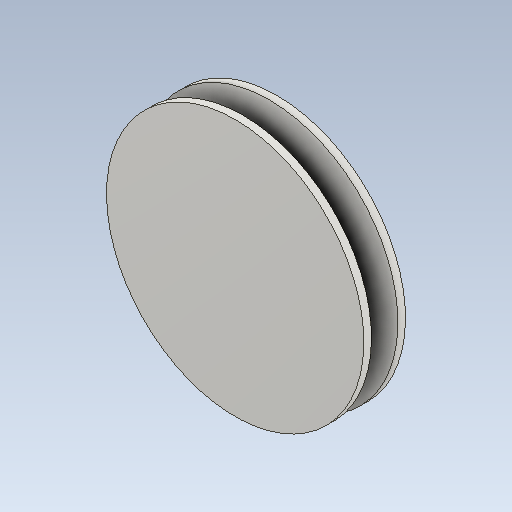
# Autodesk Inventor part: Polea ranurada1
Saved by Autodesk Inventor 2020 (Build 240168000, 168)
## iProperties
Created: 2020-12-08
Part Number: Polea ranurada1
Material: Steel
Document SubType Name: Modeling
Designer: DanielAlvaradoPelaez
Density: 1 g/cm^3
Appearance: Steel
CustomPartVersion: 1
Author: DanielAlvaradoPelaez
Autodesk Inventor part; units mm, degrees
ref_plane "YZ Plane" through (0, 0, 0) normal (1, 0, 0) x (0, 1, 0)
ref_plane "XZ Plane" through (0, 0, 0) normal (0, 1, 0) x (-1, 0, 0)
ref_plane "XY Plane" through (0, 0, 0) normal (0, 0, 1) x (1, 0, 0)
sketch "Boceto principal" plane through (0, 0, 0) normal (1, 0, 0) x (0, 1, 0)
  line L0 (0, 20) -> (61.8, 20)
  line L1 (61.8, 20) -> (61.8, 16.356)
  line L2 (61.8, 16.356) -> (48, 12.137)
  line L3 (48, 12.137) -> (48, 7.863)
  line L4 (48, 7.863) -> (61.8, 3.644)
  line L5 (61.8, 3.644) -> (61.8, 0)
  line L6 (61.8, 0) -> (0, 0)
  line L7 (59, 15.5) -> (59, 4.5) construction
  line L8 (48, 10) -> (59, 10) construction
  line L9 (61.8, 16.356) -> (61.8, 3.644)
  line L10 (0, -4) -> (0, 24) projected
  line L11 (0, 0) -> (0, 20)
  dimension "d0" = 11
  dimension "d1" = 34
  dimension "d2" = 2.8
  dimension "d6" = 20
  dimension "d21" = 118
  dimension "d25" = 13.8
  dimension "d27" = 10
  constraints: 22 end point, 5 perpendicular, 2 collinear, 2 midpoint, 2 point on line, 1 parallel
  measures "d0" distance of L7.start L7.end
  measures "d1" angle of L2 L4
  measures "d2" distance between parallel lines of L1 L7
  measures "d6" distance between parallel lines of L6 L0
  measures "d21" diameter of L7 L10
  measures "d25" distance between parallel lines of L3 L9
  measures "d27" distance between parallel lines of L6 L8
ref_plane "Plano de correa" through (0, 48, 10) normal (0, 0, 1) x (1, 0, 0)
revolve "Cuerpo" add sketch "Boceto principal" angle 360 about axis through (0, 0, -10) along (0, 0, 1)
revolve "Para ranuras" cut sketch "Boceto principal" angle 360 about axis through (0, 0, -10) along (0, 0, 1) contours L9 L4 L3 L2
fillet "Empalme externo" [suppressed]
fillet "Empalme interno" [suppressed]
pattern_of_one "Patrón para ranuras"
equation "\"d0\" = da_Bw"
equation "\"d1\" = da_Alfa"
equation "\"d2\" = da_c"
equation "\"d21\" = da_Dw"
equation "\"d25\" = da_Hd"
equation "\"d27\" = da_Se"
equation "\"da_r1\" = 0"
equation "\"da_r2\" = 0"
equation "\"d18\" = da_Sg"
equation "\"da_Bw\" = 11"
equation "\"da_Alfa\" = 34deg"
equation "\"da_c\" = 2.8"
equation "\"da_Dw\" = 118"
equation "\"da_Hd\" = 13.8"
equation "\"da_Se\" = 10"
equation "\"da_Sg\" = 15"
body "Solid1"
